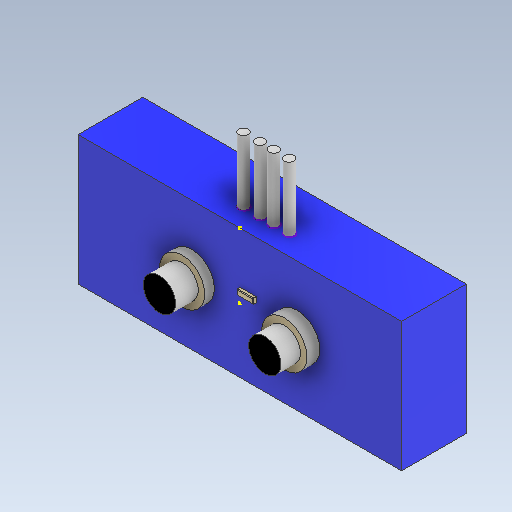
# Autodesk Inventor part: ultrasonic sensor
Saved by Autodesk Inventor 2021 (Build 250183000, 183)
## iProperties
Created: 2021-06-29
Part Number: ultrasonic sensor
Material: Generic
Document SubType Name: Modeling
Designer: HP
Density: 1 g/cm^3
Appearance: Default
Mass: 10.2987 g
Surface Area: 36.7638 cm^2
Volume: 10.2987 cm^3
Author: HP
Autodesk Inventor part; units mm, degrees
ref_plane "YZ Plane" through (0, 0, 0) normal (1, 0, 0) x (0, 1, 0)
ref_plane "XZ Plane" through (0, 0, 0) normal (0, 1, 0) x (-1, 0, 0)
ref_plane "XY Plane" through (0, 0, 0) normal (0, 0, 1) x (1, 0, 0)
sketch "Sketch1" plane through (0, 0, 0) normal (0, 0, 1) x (1, 0, 0)
  line L0 (-25, -10) -> (25, -10)
  line L1 (25, -10) -> (25, 10)
  line L2 (25, 10) -> (-25, 10)
  line L3 (-25, 10) -> (-25, -10)
  line L4 (-25, -10) -> (25, 10) construction
  line L5 (25, -10) -> (-25, 10) construction
  circle A0 centre (-7.427, -0.0759) radius 3.5
  circle A1 centre (8.8633, -0.0759) radius 3.5
  line L6 (0.033, 2.0872) -> (2.5566, 2.0872)
  line L7 (2.5566, 2.0872) -> (2.5566, 1.2559)
  line L8 (2.5566, 1.2559) -> (0.033, 1.2559)
  line L9 (0.033, 1.2559) -> (0.033, 2.0872)
  line L10 (0.033, 2.0872) -> (2.5566, 1.2559) construction
  line L11 (2.5566, 2.0872) -> (0.033, 1.2559) construction
  circle A2 centre (-7.427, -0.0759) radius 2.5
  circle A3 centre (8.8633, -0.0759) radius 2.5
  point P0 (0, 0)
  point P1 (1.2948, 1.6716)
  dimension "d0" = 7
  dimension "d1" = 7
  dimension "d11" = 5
  dimension "d12" = 5
  dimension "d28" = 50
  dimension "d29" = 20
  constraints: 24 end point, 4 centre point, 4 midpoint, 4 parallel, 2 coincident, 2 horizontal, 2 perpendicular
  measures "d0" diameter of A0
  measures "d1" diameter of A1
  measures "d11" diameter of A2
  measures "d12" diameter of A3
  measures "d28" distance of L0.start L0.end
  measures "d29" distance of L2.end L0.start
extrude "Extrusion1" add sketch "Sketch1" against normal blind 10 contours L3 L2 L1 L0 | A0 | A1 | L6 L7 L8 L9 | A2 | A3
extrude "Extrusion2" add sketch "Sketch1" along normal blind 1.5 contours A0 | A2
extrude "Extrusion3" add sketch "Sketch1" along normal blind 2 contours A1 | A3
extrude "Extrusion4" add sketch "Sketch1" along normal blind 0.5 contours L6 L7 L8 L9
fillet "Fillet1" radius 0.1 4 edges at (1.2948, 2.0872, 0.5) (2.5566, 1.6716, 0.5) (1.2948, 1.2559, 0.5) (0.033, 1.6716, 0.5)
extrude "Extrusion5" add sketch "Sketch1" along normal blind 5 contours A2
extrude "Extrusion6" add sketch "Sketch1" along normal blind 5 contours A3
sketch "Sketch3" plane through (-25, 10, 0) normal (0, 1, 0) x (1, 0, 0)
  circle A0 centre (29.4869, 3.1475) radius 0.75
  circle A1 centre (27.0793, 3.1475) radius 0.75
  circle A2 centre (25, 3.1475) radius 0.75
  circle A3 centre (22.4188, 3.1475) radius 0.75
  point P0 (25, 0)
  dimension "d19" = 1.5
  dimension "d20" = 1.5
  dimension "d21" = 1.5
  dimension "d22" = 1.5
  constraints: 4 centre point
  measures "d19" diameter of A0
  measures "d20" diameter of A1
  measures "d21" diameter of A2
  measures "d22" diameter of A3
extrude "Extrusion8" add sketch "Sketch3" along normal blind 10 contours A0 | A2 | A3
extrude "Extrusion9" add sketch "Sketch3" along normal blind 10 contours A1
sketch "Sketch4" plane through (0, 0, 0) normal (0, 0, 1) x (1, 0, 0)
  point P0 (0, 0)
body "Solid1"
